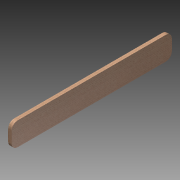
# Autodesk Inventor part: Bumper Wood Backing Part2 (26x28 robot)
Saved by Autodesk Inventor 2013 (Build 170138000, 138)
## iProperties
Created: 2013-01-06
Part Number: Bumper Wood Backing Part2 (26x28 robot)
Material: Wood (Birch)
Document SubType Name: Modeling
Designer: Moses
Density: 0.55 g/cm^3
Mass: 1156.05 g
Surface Area: 2578.08 cm^2
Volume: 2101.9 cm^3
Author: Moses
Autodesk Inventor part; units mm, degrees
ref_plane "YZ Plane" through (0, 0, 0) normal (1, 0, 0) x (0, 1, 0)
ref_plane "XZ Plane" through (0, 0, 0) normal (0, 1, 0) x (-1, 0, 0)
ref_plane "XY Plane" through (0, 0, 0) normal (0, 0, 1) x (1, 0, 0)
sketch "Sketch1" plane through (0, 0, 0) normal (0, 0, 1) x (1, 0, 0)
  line L0 (0, 0) -> (0, 127)
  line L1 (0, 127) -> (19.05, 127)
  line L2 (19.05, 127) -> (19.05, 0)
  line L3 (19.05, 0) -> (0, 0)
  dimension "d0" = 127
  dimension "d1" = 19.05
  constraints: 8 end point, 2 parallel, 1 perpendicular, 1 vertical
  measures "d0" distance of L0.start L0.end
  measures "d1" distance of L0.end L1.end
extrude "Extrusion1" add sketch "Sketch1" along normal blind 876.3
fillet "Fillet1" radius 33.3375 4 edges at (9.525, 127, 876.3) (9.525, 0, 876.3) (9.525, 127, 0) (9.525, 0, 0)
body "Solid1"
